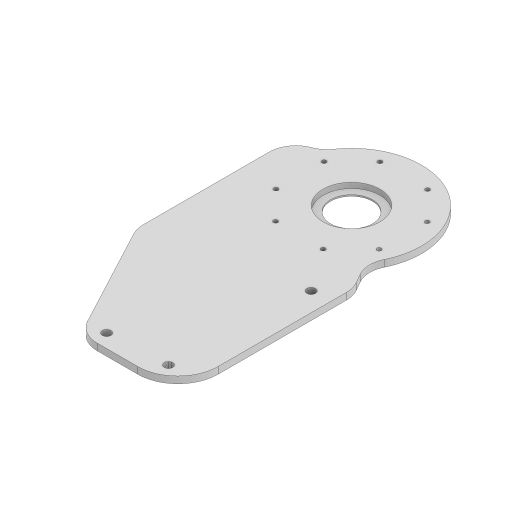
# Autodesk Inventor part: chasis lateral
Saved by Autodesk Inventor 2024.3 (Build 283343000, 343)
## iProperties
Created: 2025-10-01
Part Number: chasis lateral
Material: Generic
Document SubType Name: Modeling
Designer: danie
Density: 1 g/cm^3
Appearance: Default
Author: danie
Autodesk Inventor part; units mm, degrees
ref_plane "YZ Plane" through (0, 0, 0) normal (1, 0, 0) x (0, 1, 0)
ref_plane "XZ Plane" through (0, 0, 0) normal (0, 1, 0) x (-1, 0, 0)
ref_plane "XY Plane" through (0, 0, 0) normal (0, 0, 1) x (1, 0, 0)
sketch "Cara" plane through (0, 0, 0) normal (0, 0, 1) x (1, 0, 0)
  arc A0 (-37.5746, 19.4158) -> (-34.8255, 21.9848) centre (-41.5089, 26.3816) ccw
  arc A1 (-37.5746, 19.4158) -> (-34.8255, 21.9848) centre (-41.5089, 26.3816) ccw
  arc A2 (-40.1679, 10.4402) -> (-39.989, 14.1986) centre (-47.8453, 12.6891) ccw
  line L0 (-39.989, 14.1986) -> (-41.953, 13.8212)
  arc A3 (-41.953, 13.8212) -> (-42.0265, 14.1525) centre (-47.8453, 12.6891) ccw
  arc A4 (-40.1679, 10.4402) -> (-39.989, 14.1986) centre (-47.8453, 12.6891) ccw
  line L1 (-42.0872, 11.0024) -> (-40.1679, 10.4402)
  arc A5 (-42.0872, 11.0024) -> (-41.953, 13.8212) centre (-47.8453, 12.6891) ccw
  arc A6 (-15.0916, 39.5133) -> (-10.9897, 39.6183) centre (-13.2386, 47.2957) ccw
  arc A7 (-15.0916, 39.5133) -> (-10.9897, 39.6183) centre (-13.2386, 47.2957) ccw
  line L2 (-11.5519, 41.5377) -> (-10.9897, 39.6183)
  line L3 (-11.5519, 41.5377) -> (-10.9897, 39.6183)
  arc A8 (-14.6284, 41.4589) -> (-11.5519, 41.5377) centre (-13.2386, 47.2957) ccw
  circle A9 centre (-16.6083, 36.9072) radius 1.5875
  arc A10 (-22.3261, 34.412) -> (-19.5734, 37.455) centre (-26.6841, 41.1208) ccw
  arc A11 (-22.3261, 34.412) -> (-19.5734, 37.455) centre (-26.6841, 41.1208) ccw
  line L4 (-21.3511, 38.3714) -> (-19.5734, 37.455)
  line L5 (-21.3511, 38.3714) -> (-19.5734, 37.455)
  line L6 (-14.6284, 41.4589) -> (-15.0916, 39.5133)
  line L7 (-14.6284, 41.4589) -> (-15.0916, 39.5133)
  arc A12 (-15.0916, 39.5133) -> (-19.5734, 37.455) centre (-16.0181, 35.6221) ccw
  arc A13 (-15.0916, 39.5133) -> (-19.5734, 37.455) centre (-16.0181, 35.6221) ccw
  arc A14 (-23.4156, 36.0892) -> (-21.3511, 38.3714) centre (-26.6841, 41.1208) ccw
  arc A15 (-14.6284, 41.4589) -> (-21.3511, 38.3714) centre (-16.0181, 35.6221) ccw
  arc A16 (-38.5582, 21.1573) -> (-36.4963, 23.084) centre (-41.5089, 26.3816) ccw
  line L8 (-36.4963, 23.084) -> (-34.8255, 21.9848)
  arc A17 (-22.1052, 24.5555) -> (-22.1935, 21.6439) centre (-20.7793, 23.0582) ccw
  line L9 (-23.4156, 36.0892) -> (-22.3261, 34.412)
  line L10 (-23.4156, 36.0892) -> (-22.3261, 34.412)
  arc A18 (-22.3261, 34.412) -> (-34.8255, 21.9848) centre (1.0981, -1.6477) ccw
  arc A19 (-22.3261, 34.412) -> (-34.8255, 21.9848) centre (1.0981, -1.6477) ccw
  arc A20 (-23.4156, 36.0892) -> (-36.4963, 23.084) centre (1.0981, -1.6477) ccw
  line L11 (-36.4963, 23.084) -> (-34.8255, 21.9848)
  spline S0 degree 3 poles (-38.0493, 19.3558) (-37.9271, 19.3805) (-37.8093, 19.397) (-37.6564, 19.4108) (-37.6155, 19.4137) (-37.5746, 19.4158) knots 0 0 0 0 0.731153 0.731153 1 1 1 1
  line L12 (-38.5582, 21.1573) -> (-37.5746, 19.4158)
  line L13 (-38.5582, 21.1573) -> (-37.5746, 19.4158)
  arc A21 (-38.8583, 20.9988) -> (-38.5582, 21.1573) centre (-41.5089, 26.3816) ccw
  line L14 (-38.8583, 20.9988) -> (-38.0493, 19.3558)
  line L15 (-38.8583, 20.9988) -> (-38.0493, 19.3558)
  circle A22 centre (-37.4054, 16.1703) radius 1.5875
  arc A23 (-39.989, 14.1986) -> (-37.5746, 19.4158) centre (-37.4054, 16.1703) ccw
  circle A24 centre (-37.4054, 16.1703) radius 3.25
  spline S1 degree 3 poles (-40.2504, 14.5992) (-40.3671, 14.8104) (-40.4601, 15.0344) (-40.6458, 15.6766) (-40.6826, 16.1053) (-40.5958, 16.8869) (-40.4968, 17.2357) (-40.1864, 17.8912) (-39.9757, 18.1925) (-39.4148, 18.7612) (-39.0515, 19.0059) (-38.4565, 19.2528) (-38.255, 19.3143) (-38.0493, 19.3558) knots 0 0 0 0 0.118944 0.118944 0.328096 0.328096 0.504735 0.504735 0.683825 0.683825 0.89662 0.89662 1 1 1 1
  arc A25 (-38.8583, 20.9988) -> (-42.0265, 14.1525) centre (-36.2077, 15.616) ccw
  arc A26 (-38.8583, 20.9988) -> (-42.0265, 14.1525) centre (-36.2077, 15.616) ccw
  spline S2 degree 3 poles (-39.989, 14.1986) (-40.081, 14.3191) (-40.1695, 14.4526) (-40.2504, 14.5992) knots 0 0 0 0 1 1 1 1
  line L16 (-40.2504, 14.5992) -> (-42.0265, 14.1525)
  line L17 (-40.2504, 14.5992) -> (-42.0265, 14.1525)
  line L18 (-39.989, 14.1986) -> (-41.953, 13.8212)
  arc A27 (-9.9928, 31.5486) -> (-22.1052, 24.5555) centre (1.0981, -1.6477) ccw
  line L19 (-7.4272, 30.1693) -> (-4.8581, 20.5814)
  line L20 (-15.1747, 14.6251) -> (-22.1935, 21.6439)
  arc A28 (-6.107, 18.184) -> (-4.8581, 20.5814) centre (-6.79, 20.0638) ccw
  arc A29 (-6.107, 18.184) -> (-12.474, 14.508) centre (1.0981, -1.6477) ccw
  arc A30 (-15.1747, 14.6251) -> (-12.474, 14.508) centre (-13.7605, 16.0394) ccw
  arc A31 (12.1891, 31.5486) -> (9.6235, 30.1693) centre (11.5553, 29.6516) ccw
  arc A32 (-7.4272, 30.1693) -> (-9.9928, 31.5486) centre (-9.359, 29.6516) ccw
  arc A33 (13.186, 39.6183) -> (-10.9897, 39.6183) centre (1.0981, -1.6477) ccw
  arc A34 (13.186, 39.6183) -> (-10.9897, 39.6183) centre (1.0981, -1.6477) ccw
  arc A35 (13.7482, 41.5377) -> (-11.5519, 41.5377) centre (1.0981, -1.6477) ccw
  line L21 (13.7482, 41.5377) -> (13.186, 39.6183)
  line L22 (13.7482, 41.5377) -> (13.186, 39.6183)
  line L23 (-42.072, -17.3231) -> (-40.1338, -17.8165)
  line L24 (-42.072, -17.3231) -> (-40.1338, -17.8165)
  arc A36 (-40.1338, -17.8165) -> (-40.2027, -13.6161) centre (-47.8865, -15.8428) ccw
  arc A37 (-42.072, -17.3231) -> (-42.1236, -14.1728) centre (-47.8865, -15.8428) ccw
  line L25 (-42.1236, -14.1728) -> (-40.2027, -13.6161)
  arc A38 (-40.1338, -17.8165) -> (-40.2027, -13.6161) centre (-47.8865, -15.8428) ccw
  line L26 (-30.7188, 6.8776) -> (-21.131, 4.3086)
  arc A39 (-19.6792, 2.0283) -> (-21.131, 4.3086) centre (-21.6486, 2.3767) ccw
  arc A40 (-19.6792, 2.0283) -> (-19.6792, -5.3237) centre (1.0981, -1.6477) ccw
  arc A41 (-21.131, -7.604) -> (-19.6792, -5.3237) centre (-21.6486, -5.6721) ccw
  line L27 (-21.131, -7.604) -> (-30.7188, -10.173)
  arc A42 (-33.1961, -8.6408) -> (-30.7188, -10.173) centre (-31.2365, -8.2412) ccw
  arc A43 (-33.1961, 5.3454) -> (-33.1961, -8.6408) centre (1.0981, -1.6477) ccw
  arc A44 (-40.1679, 10.4402) -> (-40.2027, -13.6161) centre (1.0981, -1.6477) ccw
  arc A45 (-42.0872, 11.0024) -> (-42.1236, -14.1728) centre (1.0981, -1.6477) ccw
  arc A46 (-30.7188, 6.8776) -> (-33.1961, 5.3454) centre (-31.2365, 4.9458) ccw
  spline S3 degree 3 poles (22.1017, 37.4997) (22.1264, 37.3775) (22.1428, 37.2598) (22.1566, 37.1069) (22.1595, 37.0659) (22.1617, 37.0251) knots 0 0 0 0 0.731153 0.731153 1 1 1 1
  circle A47 centre (18.9161, 36.8558) radius 1.5875
  arc A48 (16.9444, 39.4394) -> (22.1617, 37.0251) centre (18.9161, 36.8558) ccw
  circle A49 centre (18.9161, 36.8558) radius 3.25
  arc A50 (13.186, 39.6183) -> (16.9444, 39.4394) centre (15.4349, 47.2957) ccw
  arc A51 (13.186, 39.6183) -> (16.9444, 39.4394) centre (15.4349, 47.2957) ccw
  spline S4 degree 3 poles (17.3451, 39.7009) (17.5563, 39.8175) (17.7803, 39.9105) (18.4224, 40.0962) (18.8512, 40.133) (19.6327, 40.0462) (19.9815, 39.9473) (20.6371, 39.6368) (20.9383, 39.4261) (21.507, 38.8652) (21.7517, 38.502) (21.9986, 37.907) (22.0601, 37.7054) (22.1017, 37.4997) knots 0 0 0 0 0.118944 0.118944 0.328096 0.328096 0.504735 0.504735 0.683825 0.683825 0.89662 0.89662 1 1 1 1
  arc A52 (23.7446, 38.3088) -> (16.8984, 41.4769) centre (18.3618, 35.6581) ccw
  spline S5 degree 3 poles (16.9444, 39.4394) (17.0649, 39.5314) (17.1985, 39.6199) (17.3451, 39.7009) knots 0 0 0 0 1 1 1 1
  arc A53 (13.7482, 41.5377) -> (16.567, 41.4035) centre (15.4349, 47.2957) ccw
  line L28 (16.9444, 39.4394) -> (16.567, 41.4035)
  line L29 (17.3451, 39.7009) -> (16.8984, 41.4769)
  line L30 (17.3451, 39.7009) -> (16.8984, 41.4769)
  arc A54 (16.567, 41.4035) -> (16.8984, 41.4769) centre (15.4349, 47.2957) ccw
  line L31 (16.9444, 39.4394) -> (16.567, 41.4035)
  circle A55 centre (-37.4568, -19.3542) radius 1.5875
  arc A56 (-42.072, -17.3231) -> (-38.9237, -24.1785) centre (-36.2575, -18.8034) ccw
  arc A57 (-40.1338, -17.8165) -> (-38.0349, -22.3868) centre (-36.2575, -18.8034) ccw
  arc A58 (-40.1338, -17.8165) -> (-38.0349, -22.3868) centre (-36.2575, -18.8034) ccw
  line L32 (-38.9237, -24.1785) -> (-38.0349, -22.3868)
  arc A59 (-36.5677, -26.2705) -> (-38.9237, -24.1785) centre (-41.5898, -29.5536) ccw
  arc A60 (-34.8937, -25.1762) -> (-38.0349, -22.3868) centre (-41.5898, -29.5536) ccw
  arc A61 (-34.8937, -25.1762) -> (-38.0349, -22.3868) centre (-41.5898, -29.5536) ccw
  line L33 (-36.5677, -26.2705) -> (-34.8937, -25.1762)
  line L34 (-36.5677, -26.2705) -> (-34.8937, -25.1762)
  line L35 (-38.9237, -24.1785) -> (-38.0349, -22.3868)
  arc A62 (22.1617, 37.0251) -> (24.7307, 34.2759) centre (29.1274, 40.9594) ccw
  line L36 (23.7446, 38.3088) -> (22.1017, 37.4997)
  line L37 (23.7446, 38.3088) -> (22.1017, 37.4997)
  arc A63 (23.7446, 38.3088) -> (23.9031, 38.0086) centre (29.1274, 40.9594) ccw
  line L38 (23.9031, 38.0086) -> (22.1617, 37.0251)
  line L39 (23.9031, 38.0086) -> (22.1617, 37.0251)
  arc A64 (22.1617, 37.0251) -> (24.7307, 34.2759) centre (29.1274, 40.9594) ccw
  line L40 (25.8298, 35.9468) -> (24.7307, 34.2759)
  line L41 (25.8298, 35.9468) -> (24.7307, 34.2759)
  arc A65 (23.9031, 38.0086) -> (25.8298, 35.9468) centre (29.1274, 40.9594) ccw
  line L42 (24.3898, 21.6439) -> (17.371, 14.6251)
  arc A66 (14.6703, 14.508) -> (17.371, 14.6251) centre (15.9568, 16.0394) ccw
  arc A67 (14.6703, 14.508) -> (8.3033, 18.184) centre (1.0981, -1.6477) ccw
  line L43 (7.0544, 20.5814) -> (9.6235, 30.1693)
  arc A68 (7.0544, 20.5814) -> (8.3033, 18.184) centre (8.9863, 20.0638) ccw
  arc A69 (24.3015, 24.5555) -> (12.1891, 31.5486) centre (1.0981, -1.6477) ccw
  arc A70 (24.3898, 21.6439) -> (24.3015, 24.5555) centre (22.9756, 23.0582) ccw
  arc A71 (37.09, 21.8808) -> (24.7307, 34.2759) centre (1.0981, -1.6477) ccw
  arc A72 (37.09, 21.8808) -> (24.7307, 34.2759) centre (1.0981, -1.6477) ccw
  arc A73 (38.764, 22.9751) -> (25.8298, 35.9468) centre (1.0981, -1.6477) ccw
  arc A74 (-22.1935, -24.9393) -> (-22.1052, -27.8509) centre (-20.7793, -26.3535) ccw
  arc A75 (-34.8937, -25.1762) -> (-22.5344, -37.5713) centre (1.0981, -1.6477) ccw
  arc A76 (-34.8937, -25.1762) -> (-22.5344, -37.5713) centre (1.0981, -1.6477) ccw
  arc A77 (-36.5677, -26.2705) -> (-23.6336, -39.2421) centre (1.0981, -1.6477) ccw
  arc A78 (-19.9654, -40.3204) -> (-22.5344, -37.5713) centre (-26.9311, -44.2547) ccw
  arc A79 (-21.5483, -41.6041) -> (-21.7068, -41.304) centre (-26.9311, -44.2547) ccw
  line L44 (-21.7068, -41.304) -> (-19.9654, -40.3204)
  line L45 (-21.7068, -41.304) -> (-19.9654, -40.3204)
  arc A80 (-19.9654, -40.3204) -> (-22.5344, -37.5713) centre (-26.9311, -44.2547) ccw
  arc A81 (-21.7068, -41.304) -> (-23.6336, -39.2421) centre (-26.9311, -44.2547) ccw
  line L46 (-23.6336, -39.2421) -> (-22.5344, -37.5713)
  line L47 (-23.6336, -39.2421) -> (-22.5344, -37.5713)
  line L48 (-4.8581, -23.8768) -> (-7.4272, -33.4646)
  arc A82 (-22.1052, -27.8509) -> (-9.9928, -34.8439) centre (1.0981, -1.6477) ccw
  line L49 (-22.1935, -24.9393) -> (-15.1747, -17.9205)
  circle A83 centre (-16.7198, -40.1512) radius 1.5875
  spline S6 degree 3 poles (-19.9054, -40.7951) (-19.9301, -40.6729) (-19.9466, -40.5552) (-19.9604, -40.4023) (-19.9633, -40.3613) (-19.9654, -40.3204) knots 0 0 0 0 0.731153 0.731153 1 1 1 1
  line L50 (-21.5483, -41.6041) -> (-19.9054, -40.7951)
  line L51 (-21.5483, -41.6041) -> (-19.9054, -40.7951)
  arc A84 (-14.7481, -42.7348) -> (-19.9654, -40.3204) centre (-16.7198, -40.1512) ccw
  circle A85 centre (-16.7198, -40.1512) radius 3.25
  spline S7 degree 3 poles (-14.7481, -42.7348) (-14.8686, -42.8268) (-15.0022, -42.9153) (-15.1488, -42.9963) knots 0 0 0 0 1 1 1 1
  spline S8 degree 3 poles (-15.1488, -42.9963) (-15.36, -43.1129) (-15.584, -43.2059) (-16.2261, -43.3916) (-16.6549, -43.4284) (-17.4365, -43.3416) (-17.7852, -43.2427) (-18.4408, -42.9322) (-18.742, -42.7215) (-19.3107, -42.1606) (-19.5554, -41.7973) (-19.8023, -41.2024) (-19.8638, -41.0008) (-19.9054, -40.7951) knots 0 0 0 0 0.118944 0.118944 0.328096 0.328096 0.504735 0.504735 0.683825 0.683825 0.89662 0.89662 1 1 1 1
  arc A86 (-21.5483, -41.6041) -> (-14.7021, -44.7723) centre (-16.1656, -38.9535) ccw
  line L52 (-14.7481, -42.7348) -> (-14.3707, -44.6989)
  line L53 (-14.7481, -42.7348) -> (-14.3707, -44.6989)
  line L54 (-15.1488, -42.9963) -> (-14.7021, -44.7723)
  line L55 (-15.1488, -42.9963) -> (-14.7021, -44.7723)
  arc A87 (-12.474, -17.8034) -> (-15.1747, -17.9205) centre (-13.7605, -19.3347) ccw
  arc A88 (-12.474, -17.8034) -> (-6.107, -21.4794) centre (1.0981, -1.6477) ccw
  arc A89 (-4.8581, -23.8768) -> (-6.107, -21.4794) centre (-6.79, -23.3592) ccw
  arc A90 (8.3033, -21.4794) -> (7.0544, -23.8768) centre (8.9863, -23.3592) ccw
  arc A91 (8.3033, -21.4794) -> (14.6703, -17.8034) centre (1.0981, -1.6477) ccw
  arc A92 (17.371, -17.9205) -> (14.6703, -17.8034) centre (15.9568, -19.3347) ccw
  circle A93 centre (1.0981, -1.6477) radius 15.5
  circle A94 centre (39.653, 16.0588) radius 1.5875
  arc A95 (42.3301, 14.5211) -> (40.2312, 19.0914) centre (38.4538, 15.508) ccw
  arc A96 (37.09, 21.8808) -> (40.2312, 19.0914) centre (43.7861, 26.2582) ccw
  line L56 (37.09, 21.8808) -> (38.764, 22.9751)
  line L57 (37.09, 21.8808) -> (38.764, 22.9751)
  arc A97 (38.764, 22.9751) -> (41.1199, 20.8831) centre (43.7861, 26.2582) ccw
  arc A98 (37.09, 21.8808) -> (40.2312, 19.0914) centre (43.7861, 26.2582) ccw
  line L58 (41.1199, 20.8831) -> (40.2312, 19.0914)
  line L59 (41.1199, 20.8831) -> (40.2312, 19.0914)
  arc A99 (42.3301, 14.5211) -> (40.2312, 19.0914) centre (38.4538, 15.508) ccw
  arc A100 (44.2683, 14.0277) -> (41.1199, 20.8831) centre (38.4538, 15.508) ccw
  line L60 (32.9151, -10.173) -> (23.3272, -7.604)
  arc A101 (21.8755, -5.3237) -> (23.3272, -7.604) centre (23.8449, -5.6721) ccw
  arc A102 (21.8755, -5.3237) -> (21.8755, 2.0283) centre (1.0981, -1.6477) ccw
  arc A103 (32.9151, -10.173) -> (35.3924, -8.6408) centre (33.4327, -8.2412) ccw
  arc A104 (35.3924, 5.3454) -> (32.9151, 6.8776) centre (33.4327, 4.9458) ccw
  line L61 (23.3272, 4.3086) -> (32.9151, 6.8776)
  arc A105 (23.3272, 4.3086) -> (21.8755, 2.0283) centre (23.8449, 2.3767) ccw
  arc A106 (35.3924, -8.6408) -> (35.3924, 5.3454) centre (1.0981, -1.6477) ccw
  circle A107 centre (39.6017, -19.4656) radius 1.5875
  arc A108 (42.1093, -17.3982) -> (39.7709, -22.7112) centre (39.6017, -19.4656) ccw
  circle A109 centre (39.6017, -19.4656) radius 3.25
  arc A110 (42.3332, -13.8408) -> (42.1093, -17.3982) centre (50.0048, -16.1093) ccw
  arc A111 (42.3332, -13.8408) -> (42.1093, -17.3982) centre (50.0048, -16.1093) ccw
  arc A112 (42.3301, 14.5211) -> (42.3989, 10.3207) centre (50.0828, 12.5474) ccw
  arc A113 (42.3301, 14.5211) -> (42.3989, 10.3207) centre (50.0828, 12.5474) ccw
  line L62 (44.2683, 14.0277) -> (42.3301, 14.5211)
  line L63 (44.2683, 14.0277) -> (42.3301, 14.5211)
  arc A114 (44.2683, 14.0277) -> (44.3199, 10.8774) centre (50.0828, 12.5474) ccw
  line L64 (44.3199, 10.8774) -> (42.3989, 10.3207)
  line L65 (44.3199, 10.8774) -> (42.3989, 10.3207)
  arc A115 (42.3332, -13.8408) -> (42.3989, 10.3207) centre (1.0981, -1.6477) ccw
  arc A116 (42.3332, -13.8408) -> (42.3989, 10.3207) centre (1.0981, -1.6477) ccw
  arc A117 (44.2511, -14.4079) -> (44.3199, 10.8774) centre (1.0981, -1.6477) ccw
  arc A118 (-9.9928, -34.8439) -> (-7.4272, -33.4646) centre (-9.359, -32.947) ccw
  arc A119 (9.6235, -33.4646) -> (12.1891, -34.8439) centre (11.5553, -32.947) ccw
  arc A120 (-10.9897, -42.9137) -> (-14.7481, -42.7348) centre (-13.2386, -50.5911) ccw
  arc A121 (-10.9897, -42.9137) -> (13.0666, -42.9485) centre (1.0981, -1.6477) ccw
  arc A122 (-10.9897, -42.9137) -> (13.0666, -42.9485) centre (1.0981, -1.6477) ccw
  arc A123 (-10.9897, -42.9137) -> (13.0666, -42.9485) centre (1.0981, -1.6477) ccw
  arc A124 (-11.5519, -44.8331) -> (13.6232, -44.8695) centre (1.0981, -1.6477) ccw
  line L66 (-11.5519, -44.8331) -> (-10.9897, -42.9137)
  line L67 (-11.5519, -44.8331) -> (-10.9897, -42.9137)
  arc A125 (-10.9897, -42.9137) -> (-14.7481, -42.7348) centre (-13.2386, -50.5911) ccw
  arc A126 (-11.5519, -44.8331) -> (-14.3707, -44.6989) centre (-13.2386, -50.5911) ccw
  arc A127 (-14.3707, -44.6989) -> (-14.7021, -44.7723) centre (-13.2386, -50.5911) ccw
  line L68 (44.2511, -14.4079) -> (42.3332, -13.8408)
  line L69 (42.4708, -17.939) -> (44.1743, -17.5253)
  line L70 (42.1093, -17.3982) -> (44.0832, -17.076)
  spline S9 degree 3 poles (42.1093, -17.3982) (42.1251, -17.4173) (42.1406, -17.4367) (42.2692, -17.6002) (42.376, -17.7609) (42.4708, -17.939) knots 0 0 0 0 0.119683 0.119683 1 1 1 1
  line L71 (42.4708, -17.939) -> (44.1743, -17.5253)
  line L72 (42.1093, -17.3982) -> (44.0832, -17.076)
  arc A128 (44.0832, -17.076) -> (44.1743, -17.5253) centre (50.0048, -16.1093) ccw
  arc A129 (44.2511, -14.4079) -> (44.0832, -17.076) centre (50.0048, -16.1093) ccw
  line L73 (44.2511, -14.4079) -> (42.3332, -13.8408)
  arc A130 (39.7709, -22.7112) -> (37.0217, -25.2802) centre (43.7052, -29.6769) ccw
  spline S10 degree 3 poles (42.4708, -17.939) (42.66, -18.2947) (42.7816, -18.6826) (42.8764, -19.4825) (42.8492, -19.8873) (42.6667, -20.5952) (42.5369, -20.899) (42.1389, -21.5409) (41.845, -21.8556) (41.1886, -22.3275) (40.8415, -22.494) (40.3834, -22.6216) (40.2925, -22.6427) (40.2009, -22.6599) knots 0 0 0 0 0.198107 0.198107 0.395669 0.395669 0.556952 0.556952 0.766408 0.766408 0.954091 0.954091 1 1 1 1
  line L74 (41.0245, -24.3091) -> (40.2009, -22.6599)
  arc A131 (41.0245, -24.3091) -> (44.1743, -17.5253) centre (38.3438, -18.9413) ccw
  spline S11 degree 3 poles (40.2009, -22.6599) (40.0946, -22.6799) (39.9919, -22.6936) (39.8527, -22.7062) (39.8117, -22.7091) (39.7709, -22.7112) knots 0 0 0 0 0.704713 0.704713 1 1 1 1
  arc A132 (41.0245, -24.3091) -> (40.7545, -24.4527) centre (43.7052, -29.6769) ccw
  line L75 (41.0245, -24.3091) -> (40.2009, -22.6599)
  line L76 (40.7545, -24.4527) -> (39.7709, -22.7112)
  arc A133 (40.7545, -24.4527) -> (38.6926, -26.3794) centre (43.7052, -29.6769) ccw
  arc A134 (39.7709, -22.7112) -> (37.0217, -25.2802) centre (43.7052, -29.6769) ccw
  line L77 (38.6926, -26.3794) -> (37.0217, -25.2802)
  line L78 (40.7545, -24.4527) -> (39.7709, -22.7112)
  line L79 (17.371, -17.9205) -> (24.3898, -24.9393)
  arc A135 (24.3015, -27.8509) -> (24.3898, -24.9393) centre (22.9756, -26.3535) ccw
  arc A136 (24.5347, -37.6994) -> (21.7574, -40.7935) centre (28.895, -44.4067) ccw
  arc A137 (24.5347, -37.6994) -> (37.0217, -25.2802) centre (1.0981, -1.6477) ccw
  arc A138 (24.5347, -37.6994) -> (37.0217, -25.2802) centre (1.0981, -1.6477) ccw
  arc A139 (25.6248, -39.3763) -> (38.6926, -26.3794) centre (1.0981, -1.6477) ccw
  line L80 (25.6248, -39.3763) -> (24.5347, -37.6994)
  line L81 (25.6248, -39.3763) -> (24.5347, -37.6994)
  arc A140 (25.6248, -39.3763) -> (23.5418, -41.6968) centre (28.895, -44.4067) ccw
  arc A141 (24.5347, -37.6994) -> (21.7574, -40.7935) centre (28.895, -44.4067) ccw
  line L82 (23.5418, -41.6968) -> (21.7574, -40.7935)
  line L83 (23.5418, -41.6968) -> (21.7574, -40.7935)
  line L84 (38.6926, -26.3794) -> (37.0217, -25.2802)
  line L85 (9.6235, -33.4646) -> (7.0544, -23.8768)
  arc A142 (12.1891, -34.8439) -> (24.3015, -27.8509) centre (1.0981, -1.6477) ccw
  circle A143 centre (18.8046, -40.2026) radius 1.5875
  arc A144 (17.2235, -42.8687) -> (13.0666, -42.9485) centre (15.2932, -50.6324) ccw
  arc A145 (17.2235, -42.8687) -> (21.7574, -40.7935) centre (18.1887, -38.9869) ccw
  arc A146 (16.7409, -44.8096) -> (23.5418, -41.6968) centre (18.1887, -38.9869) ccw
  arc A147 (17.2235, -42.8687) -> (21.7574, -40.7935) centre (18.1887, -38.9869) ccw
  line L86 (16.7409, -44.8096) -> (17.2235, -42.8687)
  line L87 (16.7409, -44.8096) -> (17.2235, -42.8687)
  arc A148 (16.7409, -44.8096) -> (13.6232, -44.8695) centre (15.2932, -50.6324) ccw
  line L88 (13.6232, -44.8695) -> (13.0666, -42.9485)
  line L89 (13.6232, -44.8695) -> (13.0666, -42.9485)
  arc A149 (17.2235, -42.8687) -> (13.0666, -42.9485) centre (15.2932, -50.6324) ccw
  point P0 (1.3022, -1.7009)
sketch "Sketch1" plane through (0, 0, 0) normal (0, 1, 0) x (-1, 0, 0)
  circle A0 centre (0, 0) radius 4.0988
  line L0 (124.0666, 265.2524) -> (124.0666, -182.0402) construction
  line L1 (124.0666, -182.0402) -> (-344.136, -182.0402) construction
  line L2 (-344.136, -182.0402) -> (-344.136, 265.2524) construction
  line L3 (-344.136, 265.2524) -> (124.0666, 265.2524) construction
  line L4 (0, 0) -> (44.9988, -0.3229) construction
  line L5 (0, 0) -> (-0.2655, -44.9992) construction
  line L6 (0, 0) -> (0.2004, 44.9996) construction
  line L7 (0, 0) -> (-40, 70)
  line L8 (0, 0) -> (65, -0.2894)
  line L9 (65, -0.2894) -> (65, 94.7106)
  line L10 (65, 94.7106) -> (17.9892, 182.9715)
  line L11 (17.9892, 182.9715) -> (-54.0108, 182.9715)
  line L12 (-54.0108, 182.9715) -> (-54.0108, 52.5186)
  line L13 (65, -0.2894) -> (65, -17.2894)
  line L14 (-54.0108, 52.5186) -> (0.5645, -42.9882)
  line L15 (65, -17.2894) -> (0.5645, -42.9882)
  circle A1 centre (0, 0) radius 52.0295
  circle A2 centre (-40, 70) radius 2
  arc A3 (-38.5786, 21.2355) -> (-35.818, 23.7922) centre (-42.4818, 28.2187) ccw
  arc A4 (-38.5786, 21.2355) -> (-35.818, 23.7922) centre (-42.4818, 28.2187) ccw
  arc A5 (-41.2118, 12.2715) -> (-41.0161, 16.029) centre (-48.8791, 14.5546) ccw
  line L16 (-41.0161, 16.029) -> (-42.9819, 15.6604)
  arc A6 (-42.9819, 15.6604) -> (-43.0538, 15.9921) centre (-48.8791, 14.5546) ccw
  arc A7 (-41.2118, 12.2715) -> (-41.0161, 16.029) centre (-48.8791, 14.5546) ccw
  line L17 (-43.1286, 12.8423) -> (-41.2118, 12.2715)
  arc A8 (-43.1286, 12.8423) -> (-42.9819, 15.6604) centre (-48.8791, 14.5546) ccw
  arc A9 (-16.0063, 41.2326) -> (-11.904, 41.3194) centre (-14.1187, 49.0068) ccw
  arc A10 (-16.0063, 41.2326) -> (-11.904, 41.3194) centre (-14.1187, 49.0068) ccw
  line L18 (-12.4577, 43.2413) -> (-11.904, 41.3194)
  line L19 (-12.4577, 43.2413) -> (-11.904, 41.3194)
  arc A11 (-15.5344, 43.1762) -> (-12.4577, 43.2413) centre (-14.1187, 49.0068) ccw
  circle A12 centre (-17.5346, 38.6334) radius 1.5875
  arc A13 (-23.2635, 36.1637) -> (-20.4973, 39.1943) centre (-27.5915, 42.8918) ccw
  arc A14 (-23.2635, 36.1637) -> (-20.4973, 39.1943) centre (-27.5915, 42.8918) ccw
  line L20 (-22.2708, 40.1187) -> (-20.4973, 39.1943)
  line L21 (-22.2708, 40.1187) -> (-20.4973, 39.1943)
  line L22 (-15.5344, 43.1762) -> (-16.0063, 41.2326)
  line L23 (-15.5344, 43.1762) -> (-16.0063, 41.2326)
  arc A15 (-16.0063, 41.2326) -> (-20.4973, 39.1943) centre (-16.9501, 37.3456) ccw
  arc A16 (-16.0063, 41.2326) -> (-20.4973, 39.1943) centre (-16.9501, 37.3456) ccw
  arc A17 (-24.3455, 37.8457) -> (-22.2708, 40.1187) centre (-27.5915, 42.8918) ccw
  arc A18 (-15.5344, 43.1762) -> (-22.2708, 40.1187) centre (-16.9501, 37.3456) ccw
  arc A19 (-39.5544, 22.9813) -> (-37.484, 24.8988) centre (-42.4818, 28.2187) ccw
  line L24 (-37.484, 24.8988) -> (-35.818, 23.7922)
  arc A20 (-23.0864, 26.3062) -> (-23.1877, 23.3951) centre (-21.7672, 24.803) ccw
  line L25 (-24.3455, 37.8457) -> (-23.2635, 36.1637)
  line L26 (-24.3455, 37.8457) -> (-23.2635, 36.1637)
  arc A21 (-23.2635, 36.1637) -> (-35.818, 23.7922) centre (0, 0) ccw
  arc A22 (-23.2635, 36.1637) -> (-35.818, 23.7922) centre (0, 0) ccw
  arc A23 (-24.3455, 37.8457) -> (-37.484, 24.8988) centre (0, 0) ccw
  line L27 (-37.484, 24.8988) -> (-35.818, 23.7922)
  spline S0 degree 3 poles (-39.0535, 21.1776) (-38.9312, 21.2018) (-38.8134, 21.2177) (-38.6604, 21.2308) (-38.6194, 21.2336) (-38.5786, 21.2355) knots 0 0 0 0 0.731153 0.731153 1 1 1 1
  line L28 (-39.5544, 22.9813) -> (-38.5786, 21.2355)
  line L29 (-39.5544, 22.9813) -> (-38.5786, 21.2355)
  arc A24 (-39.8552, 22.8242) -> (-39.5544, 22.9813) centre (-42.4818, 28.2187) ccw
  line L30 (-39.8552, 22.8242) -> (-39.0535, 21.1776)
  line L31 (-39.8552, 22.8242) -> (-39.0535, 21.1776)
  circle A25 centre (-38.4238, 17.9892) radius 1.5875
  arc A26 (-41.0161, 16.029) -> (-38.5786, 21.2355) centre (-38.4238, 17.9892) ccw
  circle A27 centre (-38.4238, 17.9892) radius 3.25
  spline S1 degree 3 poles (-41.2758, 16.4309) (-41.3915, 16.6426) (-41.4835, 16.867) (-41.6664, 17.51) (-41.7013, 17.9389) (-41.611, 18.7201) (-41.5105, 19.0684) (-41.1971, 19.7226) (-40.985, 20.0229) (-40.4216, 20.5891) (-40.0573, 20.8321) (-39.4612, 21.0764) (-39.2594, 21.137) (-39.0535, 21.1776) knots 0 0 0 0 0.118944 0.118944 0.328096 0.328096 0.504735 0.504735 0.683825 0.683825 0.89662 0.89662 1 1 1 1
  arc A28 (-39.8552, 22.8242) -> (-43.0538, 15.9921) centre (-37.2286, 17.4296) ccw
  arc A29 (-39.8552, 22.8242) -> (-43.0538, 15.9921) centre (-37.2286, 17.4296) ccw
  spline S2 degree 3 poles (-41.0161, 16.029) (-41.1076, 16.15) (-41.1955, 16.2839) (-41.2758, 16.4309) knots 0 0 0 0 1 1 1 1
  line L32 (-41.2758, 16.4309) -> (-43.0538, 15.9921)
  line L33 (-41.2758, 16.4309) -> (-43.0538, 15.9921)
  line L34 (-41.0161, 16.029) -> (-42.9819, 15.6604)
  arc A30 (-10.943, 33.2453) -> (-23.0864, 26.3062) centre (0, 0) ccw
  line L35 (-8.3836, 31.8546) -> (-5.8572, 22.2554)
  line L36 (-16.2002, 16.3451) -> (-23.1877, 23.3951)
  arc A31 (-7.1168, 19.8636) -> (-5.8572, 22.2554) centre (-7.7914, 21.7464) ccw
  arc A32 (-7.1168, 19.8636) -> (-13.5001, 16.216) centre (0, 0) ccw
  arc A33 (-16.2002, 16.3451) -> (-13.5001, 16.216) centre (-14.7797, 17.753) ccw
  arc A34 (11.2386, 33.1465) -> (8.6669, 31.7787) centre (10.5964, 31.2524) ccw
  arc A35 (-8.3836, 31.8546) -> (-10.943, 33.2453) centre (-10.3177, 31.3456) ccw
  arc A36 (12.2715, 41.2118) -> (-11.904, 41.3194) centre (0, 0) ccw
  arc A37 (12.2715, 41.2118) -> (-11.904, 41.3194) centre (0, 0) ccw
  arc A38 (12.8423, 43.1286) -> (-12.4577, 43.2413) centre (0, 0) ccw
  line L37 (12.8423, 43.1286) -> (12.2715, 41.2118)
  line L38 (12.8423, 43.1286) -> (12.2715, 41.2118)
  line L39 (-43.2395, -15.483) -> (-41.3036, -15.9851)
  line L40 (-43.2395, -15.483) -> (-41.3036, -15.9851)
  arc A39 (-41.3036, -15.9851) -> (-41.3537, -11.7844) centre (-49.0474, -13.9769) ccw
  arc A40 (-43.2395, -15.483) -> (-43.2771, -12.3325) centre (-49.0474, -13.9769) ccw
  line L41 (-43.2771, -12.3325) -> (-41.3537, -11.7844)
  arc A41 (-41.3036, -15.9851) -> (-41.3537, -11.7844) centre (-49.0474, -13.9769) ccw
  line L42 (-31.7787, 8.6669) -> (-22.2024, 6.0552)
  arc A42 (-20.7607, 3.7685) -> (-22.2024, 6.0552) centre (-22.7286, 4.1257) ccw
  arc A43 (-20.7607, 3.7685) -> (-20.7935, -3.5834) centre (0, 0) ccw
  arc A44 (-22.2554, -5.8572) -> (-20.7935, -3.5834) centre (-22.7644, -3.9231) ccw
  line L43 (-22.2554, -5.8572) -> (-31.8546, -8.3836)
  arc A45 (-34.3251, -6.8403) -> (-31.8546, -8.3836) centre (-32.3636, -6.4494) ccw
  arc A46 (-34.2628, 7.1457) -> (-34.3251, -6.8403) centre (0, 0) ccw
  arc A47 (-41.2118, 12.2715) -> (-41.3537, -11.7844) centre (0, 0) ccw
  arc A48 (-43.1286, 12.8423) -> (-43.2771, -12.3325) centre (0, 0) ccw
  arc A49 (-31.7787, 8.6669) -> (-34.2628, 7.1457) centre (-32.3049, 6.7374) ccw
  spline S3 degree 3 poles (21.1776, 39.0535) (21.2018, 38.9312) (21.2177, 38.8134) (21.2308, 38.6604) (21.2336, 38.6194) (21.2355, 38.5786) knots 0 0 0 0 0.731153 0.731153 1 1 1 1
  circle A50 centre (17.9892, 38.4238) radius 1.5875
  arc A51 (16.029, 41.0161) -> (21.2355, 38.5786) centre (17.9892, 38.4238) ccw
  circle A52 centre (17.9892, 38.4238) radius 3.25
  arc A53 (12.2715, 41.2118) -> (16.029, 41.0161) centre (14.5546, 48.8791) ccw
  arc A54 (12.2715, 41.2118) -> (16.029, 41.0161) centre (14.5546, 48.8791) ccw
  spline S4 degree 3 poles (16.4309, 41.2758) (16.6426, 41.3915) (16.867, 41.4835) (17.51, 41.6664) (17.9389, 41.7013) (18.7201, 41.611) (19.0684, 41.5105) (19.7226, 41.1971) (20.0229, 40.985) (20.5891, 40.4216) (20.8321, 40.0573) (21.0764, 39.4612) (21.137, 39.2594) (21.1776, 39.0535) knots 0 0 0 0 0.118944 0.118944 0.328096 0.328096 0.504735 0.504735 0.683825 0.683825 0.89662 0.89662 1 1 1 1
  arc A55 (22.8242, 39.8552) -> (15.9921, 43.0538) centre (17.4296, 37.2286) ccw
  spline S5 degree 3 poles (16.029, 41.0161) (16.15, 41.1076) (16.2839, 41.1955) (16.4309, 41.2758) knots 0 0 0 0 1 1 1 1
  arc A56 (12.8423, 43.1286) -> (15.6604, 42.9819) centre (14.5546, 48.8791) ccw
  line L44 (16.029, 41.0161) -> (15.6604, 42.9819)
  line L45 (16.4309, 41.2758) -> (15.9921, 43.0538)
  line L46 (16.4309, 41.2758) -> (15.9921, 43.0538)
  arc A57 (15.6604, 42.9819) -> (15.9921, 43.0538) centre (14.5546, 48.8791) ccw
  line L47 (16.029, 41.0161) -> (15.6604, 42.9819)
  circle A58 centre (-38.6334, -17.5346) radius 1.5875
  arc A59 (-43.2395, -15.483) -> (-40.1217, -22.3524) centre (-37.4316, -16.9892) ccw
  arc A60 (-41.3036, -15.9851) -> (-39.225, -20.5646) centre (-37.4316, -16.9892) ccw
  arc A61 (-41.3036, -15.9851) -> (-39.225, -20.5646) centre (-37.4316, -16.9892) ccw
  line L48 (-40.1217, -22.3524) -> (-39.225, -20.5646)
  arc A62 (-37.7751, -24.4549) -> (-40.1217, -22.3524) centre (-42.8118, -27.7155) ccw
  arc A63 (-36.0962, -23.368) -> (-39.225, -20.5646) centre (-42.8118, -27.7155) ccw
  arc A64 (-36.0962, -23.368) -> (-39.225, -20.5646) centre (-42.8118, -27.7155) ccw
  line L49 (-37.7751, -24.4549) -> (-36.0962, -23.368)
  line L50 (-37.7751, -24.4549) -> (-36.0962, -23.368)
  line L51 (-40.1217, -22.3524) -> (-39.225, -20.5646)
  arc A65 (21.2355, 38.5786) -> (23.7922, 35.818) centre (28.2187, 42.4818) ccw
  line L52 (22.8242, 39.8552) -> (21.1776, 39.0535)
  line L53 (22.8242, 39.8552) -> (21.1776, 39.0535)
  arc A66 (22.8242, 39.8552) -> (22.9813, 39.5544) centre (28.2187, 42.4818) ccw
  line L54 (22.9813, 39.5544) -> (21.2355, 38.5786)
  line L55 (22.9813, 39.5544) -> (21.2355, 38.5786)
  arc A67 (21.2355, 38.5786) -> (23.7922, 35.818) centre (28.2187, 42.4818) ccw
  line L56 (24.8988, 37.484) -> (23.7922, 35.818)
  line L57 (24.8988, 37.484) -> (23.7922, 35.818)
  arc A68 (22.9813, 39.5544) -> (24.8988, 37.484) centre (28.2187, 42.4818) ccw
  line L58 (23.3951, 23.1877) -> (16.3451, 16.2002)
  arc A69 (13.644, 16.0951) -> (16.3451, 16.2002) centre (14.9372, 17.6207) ccw
  arc A70 (13.644, 16.0951) -> (7.2934, 19.7994) centre (0, 0) ccw
  line L59 (6.0552, 22.2024) -> (8.6669, 31.7787)
  arc A71 (6.0552, 22.2024) -> (7.2934, 19.7994) centre (7.9847, 21.6761) ccw
  arc A72 (23.3198, 26.0996) -> (11.2386, 33.1465) centre (0, 0) ccw
  arc A73 (23.3951, 23.1877) -> (23.3198, 26.0996) centre (21.9872, 24.6082) ccw
  arc A74 (36.0962, 23.368) -> (23.7922, 35.818) centre (0, 0) ccw
  arc A75 (36.0962, 23.368) -> (23.7922, 35.818) centre (0, 0) ccw
  arc A76 (37.7751, 24.4549) -> (24.8988, 37.484) centre (0, 0) ccw
  arc A77 (-23.3951, -23.1877) -> (-23.3198, -26.0996) centre (-21.9872, -24.6082) ccw
  arc A78 (-36.0962, -23.368) -> (-23.7922, -35.818) centre (0, 0) ccw
  arc A79 (-36.0962, -23.368) -> (-23.7922, -35.818) centre (0, 0) ccw
  arc A80 (-37.7751, -24.4549) -> (-24.8988, -37.484) centre (0, 0) ccw
  arc A81 (-21.2355, -38.5786) -> (-23.7922, -35.818) centre (-28.2187, -42.4818) ccw
  arc A82 (-22.8242, -39.8552) -> (-22.9813, -39.5544) centre (-28.2187, -42.4818) ccw
  line L60 (-22.9813, -39.5544) -> (-21.2355, -38.5786)
  line L61 (-22.9813, -39.5544) -> (-21.2355, -38.5786)
  arc A83 (-21.2355, -38.5786) -> (-23.7922, -35.818) centre (-28.2187, -42.4818) ccw
  arc A84 (-22.9813, -39.5544) -> (-24.8988, -37.484) centre (-28.2187, -42.4818) ccw
  line L62 (-24.8988, -37.484) -> (-23.7922, -35.818)
  line L63 (-24.8988, -37.484) -> (-23.7922, -35.818)
  line L64 (-6.0552, -22.2024) -> (-8.6669, -31.7787)
  arc A85 (-23.3198, -26.0996) -> (-11.2386, -33.1465) centre (0, 0) ccw
  line L65 (-23.3951, -23.1877) -> (-16.3451, -16.2002)
  circle A86 centre (-17.9892, -38.4238) radius 1.5875
  spline S6 degree 3 poles (-21.1776, -39.0535) (-21.2018, -38.9312) (-21.2177, -38.8134) (-21.2308, -38.6604) (-21.2336, -38.6194) (-21.2355, -38.5786) knots 0 0 0 0 0.731153 0.731153 1 1 1 1
  line L66 (-22.8242, -39.8552) -> (-21.1776, -39.0535)
  line L67 (-22.8242, -39.8552) -> (-21.1776, -39.0535)
  arc A87 (-16.029, -41.0161) -> (-21.2355, -38.5786) centre (-17.9892, -38.4238) ccw
  circle A88 centre (-17.9892, -38.4238) radius 3.25
  spline S7 degree 3 poles (-16.029, -41.0161) (-16.15, -41.1076) (-16.2839, -41.1955) (-16.4309, -41.2758) knots 0 0 0 0 1 1 1 1
  spline S8 degree 3 poles (-16.4309, -41.2758) (-16.6426, -41.3915) (-16.867, -41.4835) (-17.51, -41.6664) (-17.9389, -41.7013) (-18.7201, -41.611) (-19.0684, -41.5105) (-19.7226, -41.1971) (-20.0229, -40.985) (-20.5891, -40.4216) (-20.8321, -40.0573) (-21.0764, -39.4612) (-21.137, -39.2594) (-21.1776, -39.0535) knots 0 0 0 0 0.118944 0.118944 0.328096 0.328096 0.504735 0.504735 0.683825 0.683825 0.89662 0.89662 1 1 1 1
  arc A89 (-22.8242, -39.8552) -> (-15.9921, -43.0538) centre (-17.4296, -37.2286) ccw
  line L68 (-16.029, -41.0161) -> (-15.6604, -42.9819)
  line L69 (-16.029, -41.0161) -> (-15.6604, -42.9819)
  line L70 (-16.4309, -41.2758) -> (-15.9921, -43.0538)
  line L71 (-16.4309, -41.2758) -> (-15.9921, -43.0538)
  arc A90 (-13.644, -16.0951) -> (-16.3451, -16.2002) centre (-14.9372, -17.6207) ccw
  arc A91 (-13.644, -16.0951) -> (-7.2934, -19.7994) centre (0, 0) ccw
  arc A92 (-6.0552, -22.2024) -> (-7.2934, -19.7994) centre (-7.9847, -21.6761) ccw
  arc A93 (7.1168, -19.8636) -> (5.8572, -22.2554) centre (7.7914, -21.7464) ccw
  arc A94 (7.1168, -19.8636) -> (13.5001, -16.216) centre (0, 0) ccw
  arc A95 (16.2002, -16.3451) -> (13.5001, -16.216) centre (14.7797, -17.753) ccw
  circle A96 centre (0, 0) radius 15.5
  circle A97 centre (38.6334, 17.5346) radius 1.5875
  arc A98 (41.3036, 15.9851) -> (39.225, 20.5646) centre (37.4316, 16.9892) ccw
  arc A99 (36.0962, 23.368) -> (39.225, 20.5646) centre (42.8118, 27.7155) ccw
  line L72 (36.0962, 23.368) -> (37.7751, 24.4549)
  line L73 (36.0962, 23.368) -> (37.7751, 24.4549)
  arc A100 (37.7751, 24.4549) -> (40.1217, 22.3524) centre (42.8118, 27.7155) ccw
  arc A101 (36.0962, 23.368) -> (39.225, 20.5646) centre (42.8118, 27.7155) ccw
  line L74 (40.1217, 22.3524) -> (39.225, 20.5646)
  line L75 (40.1217, 22.3524) -> (39.225, 20.5646)
  arc A102 (41.3036, 15.9851) -> (39.225, 20.5646) centre (37.4316, 16.9892) ccw
  arc A103 (43.2395, 15.483) -> (40.1217, 22.3524) centre (37.4316, 16.9892) ccw
  line L76 (31.7787, -8.6669) -> (22.2024, -6.0552)
  arc A104 (20.7607, -3.7685) -> (22.2024, -6.0552) centre (22.7286, -4.1257) ccw
  arc A105 (20.7607, -3.7685) -> (20.7935, 3.5834) centre (0, 0) ccw
  arc A106 (31.7787, -8.6669) -> (34.2628, -7.1457) centre (32.3049, -6.7374) ccw
  arc A107 (34.3251, 6.8403) -> (31.8546, 8.3836) centre (32.3636, 6.4494) ccw
  line L77 (22.2554, 5.8572) -> (31.8546, 8.3836)
  arc A108 (22.2554, 5.8572) -> (20.7935, 3.5834) centre (22.7644, 3.9231) ccw
  arc A109 (34.2628, -7.1457) -> (34.3251, 6.8403) centre (0, 0) ccw
  circle A110 centre (38.4238, -17.9892) radius 1.5875
  arc A111 (40.9406, -15.933) -> (38.5786, -21.2355) centre (38.4238, -17.9892) ccw
  circle A112 centre (38.4238, -17.9892) radius 3.25
  arc A113 (41.1803, -12.3766) -> (40.9406, -15.933) centre (48.8418, -14.6792) ccw
  arc A114 (41.1803, -12.3766) -> (40.9406, -15.933) centre (48.8418, -14.6792) ccw
  arc A115 (41.3036, 15.9851) -> (41.3537, 11.7844) centre (49.0474, 13.9769) ccw
  arc A116 (41.3036, 15.9851) -> (41.3537, 11.7844) centre (49.0474, 13.9769) ccw
  line L78 (43.2395, 15.483) -> (41.3036, 15.9851)
  line L79 (43.2395, 15.483) -> (41.3036, 15.9851)
  arc A117 (43.2395, 15.483) -> (43.2771, 12.3325) centre (49.0474, 13.9769) ccw
  line L80 (43.2771, 12.3325) -> (41.3537, 11.7844)
  line L81 (43.2771, 12.3325) -> (41.3537, 11.7844)
  arc A118 (41.1803, -12.3766) -> (41.3537, 11.7844) centre (0, 0) ccw
  arc A119 (41.1803, -12.3766) -> (41.3537, 11.7844) centre (0, 0) ccw
  arc A120 (43.0957, -12.9523) -> (43.2771, 12.3325) centre (0, 0) ccw
  arc A121 (-11.2386, -33.1465) -> (-8.6669, -31.7787) centre (-10.5964, -31.2524) ccw
  arc A122 (8.3836, -31.8546) -> (10.943, -33.2453) centre (10.3177, -31.3456) ccw
  arc A123 (-12.2715, -41.2118) -> (-16.029, -41.0161) centre (-14.5546, -48.8791) ccw
  arc A124 (-12.2715, -41.2118) -> (11.7844, -41.3537) centre (0, 0) ccw
  arc A125 (-12.2715, -41.2118) -> (11.7844, -41.3537) centre (0, 0) ccw
  arc A126 (-12.2715, -41.2118) -> (11.7844, -41.3537) centre (0, 0) ccw
  arc A127 (-12.8423, -43.1286) -> (12.3325, -43.2771) centre (0, 0) ccw
  line L82 (-12.8423, -43.1286) -> (-12.2715, -41.2118)
  line L83 (-12.8423, -43.1286) -> (-12.2715, -41.2118)
  arc A128 (-12.2715, -41.2118) -> (-16.029, -41.0161) centre (-14.5546, -48.8791) ccw
  arc A129 (-12.8423, -43.1286) -> (-15.6604, -42.9819) centre (-14.5546, -48.8791) ccw
  arc A130 (-15.6604, -42.9819) -> (-15.9921, -43.0538) centre (-14.5546, -48.8791) ccw
  line L84 (43.0957, -12.9523) -> (41.1803, -12.3766)
  line L85 (41.2997, -16.4754) -> (43.005, -16.0692)
  line L86 (40.9406, -15.933) -> (42.9159, -15.6196)
  spline S9 degree 3 poles (40.9406, -15.933) (40.9563, -15.9522) (40.9718, -15.9716) (41.0997, -16.1356) (41.2057, -16.2969) (41.2997, -16.4754) knots 0 0 0 0 0.119683 0.119683 1 1 1 1
  line L87 (41.2997, -16.4754) -> (43.005, -16.0692)
  line L88 (40.9406, -15.933) -> (42.9159, -15.6196)
  arc A131 (42.9159, -15.6196) -> (43.005, -16.0692) centre (48.8418, -14.6792) ccw
  arc A132 (43.0957, -12.9523) -> (42.9159, -15.6196) centre (48.8418, -14.6792) ccw
  line L89 (43.0957, -12.9523) -> (41.1803, -12.3766)
  arc A133 (38.5786, -21.2355) -> (35.818, -23.7922) centre (42.4818, -28.2187) ccw
  spline S10 degree 3 poles (41.2997, -16.4754) (41.4874, -16.8319) (41.6072, -17.2204) (41.6984, -18.0206) (41.6695, -18.4253) (41.4838, -19.1324) (41.3527, -19.4357) (40.9518, -20.0758) (40.6564, -20.3891) (39.998, -20.8581) (39.6502, -21.0231) (39.1915, -21.1486) (39.1004, -21.1694) (39.0088, -21.1861) knots 0 0 0 0 0.198107 0.198107 0.395669 0.395669 0.556952 0.556952 0.766408 0.766408 0.954091 0.954091 1 1 1 1
  line L90 (39.825, -22.839) -> (39.0088, -21.1861)
  arc A134 (39.825, -22.839) -> (43.005, -16.0692) centre (37.1682, -17.4592) ccw
  spline S11 degree 3 poles (39.0088, -21.1861) (38.9024, -21.2056) (38.7997, -21.2189) (38.6604, -21.2308) (38.6194, -21.2336) (38.5786, -21.2355) knots 0 0 0 0 0.704713 0.704713 1 1 1 1
  arc A135 (39.825, -22.839) -> (39.5544, -22.9813) centre (42.4818, -28.2187) ccw
  line L91 (39.825, -22.839) -> (39.0088, -21.1861)
  line L92 (39.5544, -22.9813) -> (38.5786, -21.2355)
  arc A136 (39.5544, -22.9813) -> (37.484, -24.8988) centre (42.4818, -28.2187) ccw
  arc A137 (38.5786, -21.2355) -> (35.818, -23.7922) centre (42.4818, -28.2187) ccw
  line L93 (37.484, -24.8988) -> (35.818, -23.7922)
  line L94 (39.5544, -22.9813) -> (38.5786, -21.2355)
  line L95 (16.2002, -16.3451) -> (23.1877, -23.3951)
  arc A138 (23.0864, -26.3062) -> (23.1877, -23.3951) centre (21.7672, -24.803) ccw
  arc A139 (23.2758, -36.1557) -> (20.4848, -39.2374) centre (27.6062, -42.8824) ccw
  arc A140 (23.2758, -36.1557) -> (35.818, -23.7922) centre (0, 0) ccw
  arc A141 (23.2758, -36.1557) -> (35.818, -23.7922) centre (0, 0) ccw
  arc A142 (24.3584, -37.8374) -> (37.484, -24.8988) centre (0, 0) ccw
  line L96 (24.3584, -37.8374) -> (23.2758, -36.1557)
  line L97 (24.3584, -37.8374) -> (23.2758, -36.1557)
  arc A143 (24.3584, -37.8374) -> (22.2651, -40.1487) centre (27.6062, -42.8824) ccw
  arc A144 (23.2758, -36.1557) -> (20.4848, -39.2374) centre (27.6062, -42.8824) ccw
  line L98 (22.2651, -40.1487) -> (20.4848, -39.2374)
  line L99 (22.2651, -40.1487) -> (20.4848, -39.2374)
  line L100 (37.484, -24.8988) -> (35.818, -23.7922)
  line L101 (8.3836, -31.8546) -> (5.8572, -22.2554)
  arc A145 (10.943, -33.2453) -> (23.0864, -26.3062) centre (0, 0) ccw
  circle A146 centre (17.5346, -38.6334) radius 1.5875
  arc A147 (15.9417, -41.2924) -> (11.7844, -41.3537) centre (13.9769, -49.0474) ccw
  arc A148 (15.9417, -41.2924) -> (20.4848, -39.2374) centre (16.9241, -37.415) ccw
  arc A149 (15.4505, -43.2312) -> (22.2651, -40.1487) centre (16.9241, -37.415) ccw
  arc A150 (15.9417, -41.2924) -> (20.4848, -39.2374) centre (16.9241, -37.415) ccw
  line L102 (15.4505, -43.2312) -> (15.9417, -41.2924)
  line L103 (15.4505, -43.2312) -> (15.9417, -41.2924)
  arc A151 (15.4505, -43.2312) -> (12.3325, -43.2771) centre (13.9769, -49.0474) ccw
  line L104 (12.3325, -43.2771) -> (11.7844, -41.3537)
  line L105 (12.3325, -43.2771) -> (11.7844, -41.3537)
  arc A152 (15.9417, -41.2924) -> (11.7844, -41.3537) centre (13.9769, -49.0474) ccw
  point P0 (45.6193, -25.019)
  point P1 (-41.7456, 31.0545)
  point P2 (-41.0161, 16.029)
  point P3 (-39.0535, 21.1776)
  dimension "d18" = 30
  dimension "d19" = 40
  dimension "d22" = 70
  dimension "d24" = 90
  dimension "d25" = 65
  dimension "d26" = 95
  dimension "d27" = 100
  dimension "d28" = 72
  dimension "d29" = 17
  dimension "d30" = 110
  dimension "d36" = 4
  constraints: 24 end point, 3 centre point, 3 coincident, 2 perpendicular, 2 vertical, 1 parallel, 6 other
  measures "d18" angle of L7 L6
  measures "d19" horizontal distance of L4.start L7.end
  measures "d22" vertical distance of L4.start L7.end
  measures "d24" angle of L6 L8
  measures "d25" horizontal distance of L4.start L8.end
  measures "d26" distance of L8.end L9.end
  measures "d27" distance of L9.end L10.end
  measures "d28" distance of L10.end L11.end
  measures "d29" distance of L8.end L13.end
  measures "d30" distance of L12.end L14.end
  measures "d36" diameter of A2
extrude "Extrusion1" add sketch "Sketch1" along normal blind 5 contours A96 L8 A105 A104 L76 A106 A109 A118 A113 A111 A133 A140 L15 L14 L64 A92 A91 A90 A44 A43 A42 L42 A3 A21 A13 L7 A30 A20 L36 A33 A32 | L7 A32 A31 L35 A35 A30 A13 A15 A9 A36 A53 A51 A65 A74 A99 A98 A115 A118 L8 A109 A107 L77 A108 A105 A96 | A32 A33 L36 A20 A30 L7 | L7 A30 A35 L35 A31 A32 | A105 A108 L77 A107 A109 L8 | L8 A109 A106 L76 A104 A105 | A13 L25 A17 L7 | L7 A17 L20 A13 | A118 L80 A120 L8 | L8 A120 L84 A118 | A17 A23 A19 L14 A1 L7 | L7 A1 L8 A120 A117 A103 A100 A76 A68 A66 A55 A57 A56 A38 A11 A18 A17 | A21 L24 A23 L25 | L20 A18 L22 A15 | L8 A1 L15 A142 A136 A135 A134 A131 A132 A120 | L84 A132 L86 A113 | A115 L78 A117 L80 | A1 L14 L12 L11 L10 L9 L8 | A3 L14 A19 L24 | L22 A11 L18 A9 | L8 L13 L15 A1 | A112 A111 | L86 A131 L85 A112 | A98 L74 A103 L78 | L14 A19 A24 A28 A6 A8 A48 A40 A59 A62 A80 A84 A82 A89 A130 A129 A127 A151 A149 A143 A142 L15 A1 | A3 L28 A19 L14 | L14 L42 A49 A46 A45 L43 A44 A90 L65 A77 A85 A121 L64 L15 A140 A139 A148 A147 A124 A123 A87 A81 A78 A63 A60 A39 A47 A5 A26 A3 | L18 A38 L37 A36 | L92 A136 L93 A133 | A112 L90 A135 L92 | L85 A134 L90 A112 | A99 L72 A100 L74 | L42 A42 A43 A44 L14 | L14 A44 L43 A45 A46 A49 L42 | A26 A27 S0 | S0 L30 A24 L28 | L37 A56 L44 A53 | A142 L96 A140 L15 | L15 A140 L93 A142 | A74 L56 A76 L72 | A27 L32 A28 L30 | A52 S3 A51 | L44 A57 L45 A52 | A143 L98 A139 L96 | A65 L54 A68 L56 | A90 A91 A92 L64 L14 | L14 L64 A121 A85 A77 L65 A90 | A27 L16 A6 L32 | A5 L17 A8 L16 | L45 A55 L52 A52 | A149 L102 A148 L98 | S3 L52 A66 L54 | A47 L41 A48 L17 | A151 L104 A147 L102 | A39 L39 A40 L41 | A127 L82 A124 L104 | A60 L48 A59 L39 | A129 L68 A123 L82 | A63 L49 A62 L48 | A130 L70 A88 L68 | A78 L62 A80 L49 | A88 S6 A87 | A89 L66 A88 L70 | A81 L60 A84 L62 | A82 L60 S6 L66 | A2 | A72 A73 L58 A69 A70 A71 L59 A34 | A94 A95 L95 A138 A145 A122 L101 A93
fillet "Fillet1" radius 30 1 edges at (54.0108, 2.5, 182.9715)
fillet "Fillet2" radius 20 1 edges at (-17.9892, 2.5, 182.9715)
fillet "Fillet3" radius 20 5 edges at (-65, 2.5, 94.7106) (-65, 2.5, -17.2894) (-45.6193, 2.5, -25.019) (54.0108, 2.5, 52.5186) (41.7456, 2.5, 31.0545)
hole "Hole1" at (40, 0, 70) direction (0, 1, 0) diameter 6.35 end through all
sketch "Sketch2" plane through (0, 5, 0) normal (0, 1, 0) x (1, 0, 0)
  circle A0 centre (40, -70) radius 3.175 projected
  arc A1 (-52.4091, 22.3111) -> (-65, 3.734) centre (-45, 3.734) ccw projected
  line L0 (-65, 3.734) -> (-65, -89.7164) projected
  arc A2 (-65, -89.7164) -> (-62.6522, -99.1185) centre (-45, -89.7164) ccw projected
  line L1 (-62.6522, -99.1185) -> (-23.634, -172.3736) projected
  arc A3 (-23.634, -172.3736) -> (-5.9818, -182.9715) centre (-5.9818, -162.9715) ccw projected
  line L2 (-5.9818, -182.9715) -> (24.0108, -182.9715) projected
  arc A4 (24.0108, -182.9715) -> (54.0108, -152.9715) centre (24.0108, -152.9715) ccw projected
  line L3 (54.0108, -152.9715) -> (54.0108, -57.8299) projected
  arc A5 (54.0108, -57.8299) -> (51.3757, -47.9071) centre (34.0108, -57.8299) ccw projected
  line L4 (51.3757, -47.9071) -> (47.5303, -41.1777) projected
  arc A6 (46.8761, -22.5766) -> (47.5303, -41.1777) centre (64.8952, -31.255) ccw projected
  arc A7 (46.8761, -22.5766) -> (-42.691, 29.7415) centre (0, 0) ccw projected
  arc A8 (-51.6922, 22.597) -> (-42.691, 29.7415) centre (-59.1013, 41.174) ccw projected
  line L5 (-51.6922, 22.597) -> (-52.4091, 22.3111) projected
  circle A9 centre (-38.4238, 17.9892) radius 1.5875 projected
  circle A10 centre (-17.9892, -38.4238) radius 1.5875 projected
  circle A11 centre (-38.6334, -17.5346) radius 1.5875 projected
  circle A12 centre (17.5346, -38.6334) radius 1.5875 projected
  circle A13 centre (-17.5346, 38.6334) radius 1.5875 projected
  circle A14 centre (38.6334, 17.5346) radius 1.5875 projected
  circle A15 centre (0, 0) radius 15.5 projected
  circle A16 centre (17.9892, 38.4238) radius 1.5875 projected
  circle A17 centre (38.4238, -17.9892) radius 1.5875 projected
  circle A18 centre (-8.9173, -172.9715) radius 3.175
  dimension "d48" = 6.35
  dimension "d49" = 10
  constraints: 1 centre point
  measures "d48" diameter of A18
  measures "d49" vertical distance of L2.start A18.centre
extrude "Extrusion2" cut sketch "Sketch2" against normal blind 5 contours A18
sketch "Sketch3" plane through (0, 5, 0) normal (0, 1, 0) x (1, 0, 0)
  circle A0 centre (-8.9173, -172.9715) radius 3.175 projected
  circle A1 centre (40, -70) radius 3.175 projected
  arc A2 (-52.4091, 22.3111) -> (-65, 3.734) centre (-45, 3.734) ccw projected
  line L0 (-65, 3.734) -> (-65, -89.7164) projected
  arc A3 (-65, -89.7164) -> (-62.6522, -99.1185) centre (-45, -89.7164) ccw projected
  line L1 (-62.6522, -99.1185) -> (-23.634, -172.3736) projected
  arc A4 (-23.634, -172.3736) -> (-5.9818, -182.9715) centre (-5.9818, -162.9715) ccw projected
  line L2 (-5.9818, -182.9715) -> (24.0108, -182.9715) projected
  arc A5 (24.0108, -182.9715) -> (54.0108, -152.9715) centre (24.0108, -152.9715) ccw projected
  line L3 (54.0108, -152.9715) -> (54.0108, -57.8299) projected
  arc A6 (54.0108, -57.8299) -> (51.3757, -47.9071) centre (34.0108, -57.8299) ccw projected
  line L4 (51.3757, -47.9071) -> (47.5303, -41.1777) projected
  arc A7 (46.8761, -22.5766) -> (47.5303, -41.1777) centre (64.8952, -31.255) ccw projected
  arc A8 (46.8761, -22.5766) -> (-42.691, 29.7415) centre (0, 0) ccw projected
  arc A9 (-51.6922, 22.597) -> (-42.691, 29.7415) centre (-59.1013, 41.174) ccw projected
  line L5 (-51.6922, 22.597) -> (-52.4091, 22.3111) projected
  circle A10 centre (-38.4238, 17.9892) radius 1.5875 projected
  circle A11 centre (-17.9892, -38.4238) radius 1.5875 projected
  circle A12 centre (-38.6334, -17.5346) radius 1.5875 projected
  circle A13 centre (17.5346, -38.6334) radius 1.5875 projected
  circle A14 centre (-17.5346, 38.6334) radius 1.5875 projected
  circle A15 centre (38.6334, 17.5346) radius 1.5875 projected
  circle A16 centre (0, 0) radius 15.5 projected
  circle A17 centre (17.9892, 38.4238) radius 1.5875 projected
  circle A18 centre (38.4238, -17.9892) radius 1.5875 projected
  line L6 (-20.9862, -170.9633) -> (-60.0044, -97.7082)
  arc A19 (-62, -89.7164) -> (-60.0044, -97.7082) centre (-45, -89.7164) ccw
  line L7 (-62, -89.7164) -> (-62, 3.734)
  arc A20 (-51.2977, 19.5245) -> (-62, 3.734) centre (-45, 3.734) ccw
  line L8 (-51.2977, 19.5245) -> (-50.5808, 19.8104)
  arc A21 (-50.5808, 19.8104) -> (-40.2294, 28.0266) centre (-59.1013, 41.174) ccw
  arc A22 (44.1733, -21.2748) -> (-40.2294, 28.0266) centre (0, 0) ccw
  arc A23 (44.1733, -21.2748) -> (44.9256, -42.6662) centre (64.8952, -31.255) ccw
  line L9 (44.9256, -42.6662) -> (48.7709, -49.3955)
  arc A24 (51.0108, -57.8299) -> (48.7709, -49.3955) centre (34.0108, -57.8299) ccw
  line L10 (51.0108, -57.8299) -> (51.0108, -152.9715)
  arc A25 (24.0108, -179.9715) -> (51.0108, -152.9715) centre (24.0108, -152.9715) ccw
  line L11 (24.0108, -179.9715) -> (-5.9818, -179.9715)
  arc A26 (-20.9862, -170.9633) -> (-5.9818, -179.9715) centre (-5.9818, -162.9715) ccw
  line L12 (-8.9173, -172.9715) -> (-8.9173, -182.7549)
  line L13 (34.6283, -170.6189) -> (39.5739, -178.6189)
  circle A27 centre (-8.9173, -182.7549) radius 15
  circle A28 centre (39.5739, -178.6189) radius 12.5
  circle A29 centre (34.6283, -170.6189) radius 3.175
  point P0 (33.7104, -167.5794)
  point P1 (32.3198, -168.4391)
  dimension "d54" = 3
  dimension "d55" = 30
  dimension "d56" = 25
  dimension "d57" = 8
  dimension "d58" = 6.35
  constraints: 18 point on circle, 16 end point, 11 centre point, 3 coincident, 1 vertical, 13 other
  measures "d54" distance between parallel lines of L1 L6
  measures "d55" diameter of A27
  measures "d56" diameter of A28
  measures "d57" vertical distance of L13.start L13.end
  measures "d58" diameter of A29
extrude "Extrusion3" cut sketch "Sketch3" against normal blind 5 contours A28 A29 picked at (34.8921, -171.697)
sketch "Sketch4" plane through (0, 5, 0) normal (0, 1, 0) x (1, 0, 0)
  circle A0 centre (0, 0) radius 21.1
  dimension "d61" = 42.2
  constraints: 1 centre point, 1 coincident
  measures "d61" diameter of A0
extrude "Extrusion4" cut sketch "Sketch4" against normal blind 4
body "Solid1"
